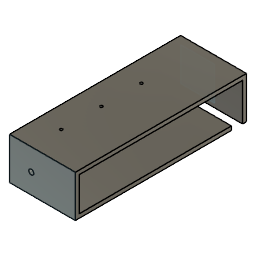
Final_3d_Model 1 (Autodesk Fusion 360 design; units mm, degrees)
part number: 2026-03-23-13-58-40-375
Autodesk Fusion 360 part; units mm, degrees
sketch "Sketch1" plane through (0, 0, 0) normal (0, 1, 0) x (1, 0, 0)
  line L0 (0, 0) -> (0, -42.3)
  line L1 (0, -42.3) -> (-42.3, -42.3)
  line L2 (-42.3, -42.3) -> (-42.3, 0)
  line L3 (-42.3, 0) -> (0, 0)
  line L4 (-42.3, -42.3) -> (-42.3, -52.3)
  line L5 (-42.3, -52.3) -> (-52.3, -52.3)
  line L6 (-52.3, -52.3) -> (10, -52.3)
  line L7 (10, -52.3) -> (10, 10)
  line L8 (10, 10) -> (-52.3, 10)
  line L9 (-52.3, 10) -> (-52.3, -52.3)
  dimension "d1" = 42.3
  dimension "d2" = 42.3
  dimension "d3" = 10
  dimension "d4" = 10
  constraint coincident L0.start L3.end
  constraint vertical L0
  constraint perpendicular L0 L1
  constraint perpendicular L1 L2
  constraint perpendicular L0 L3
  constraint perpendicular L1 L4
  constraint perpendicular L4 L5
  constraint horizontal L6
  constraint vertical L7
  constraint horizontal L8
  constraint vertical L9
  measures "d1" distance of L0.start L0.end
  measures "d2" distance of L0.end L1.end
  measures "d3" distance of L1.end L4.end
  measures "d4" distance of L4.end L5.end
extrude "Extrude1" add sketch "Sketch1" along normal blind 38.8 makes body 1
sketch "Sketch2" plane through (0, 0, 0) normal (0, 1, 0) x (1, 0, 0)
extrude "Extrude2" add 1 faces at (-28.2, 38.8, -6.6667) along direction (0, 1, 0) blind 10 on bodies 1 bodies 1
sketch "Sketch3" plane through (0, 0, 0) normal (0, 0, 1) x (-1, 0, 0)
  line L0 (42.3, 0) -> (0, 0)
  line L1 (0, 0) -> (0, -48.8)
  line L2 (0, -48.8) -> (42.3, -48.8)
  line L3 (42.3, -48.8) -> (42.3, 0)
  line L4 (42.3, -48.8) -> (0, -48.8)
  line L5 (0, -48.8) -> (0, -38.8)
  line L6 (0, -38.8) -> (42.3, -38.8)
  line L7 (42.3, -38.8) -> (42.3, -48.8)
  dimension "d9" = 10
  constraint horizontal L4
  constraint vertical L5
  constraint horizontal L6
  constraint vertical L7
  constraint coincident L2.end L3.start
  measures "d9" distance of L2.end L6.end
extrude "Extrude3" add sketch "Sketch3" along normal blind 52.3 contours L1 L2 L3 L4 L5 L6 L7 bodies 1
sketch "Sketch4" plane through (0, 38.8, 0) normal (0, -1, 0) x (1, 0, 0)
  line L0 (0, 42.3) -> (-42.3, 42.3)
  line L1 (-42.3, 42.3) -> (-42.3, 0)
  line L2 (-42.3, 0) -> (0, 0)
  line L3 (0, 0) -> (0, 42.3)
sketch "Sketch5" plane through (0, 0, 0) normal (0, 1, 0) x (1, 0, 0)
  circle A0 centre (-20, -20) radius 3
  dimension "d12" = 6
  measures "d12" diameter of A0
extrude "Extrude4" add sketch "Sketch5" against normal blind 250 separate body makes body 2
sketch "Sketch6" plane through (0, 0, 0) normal (0, 1, 0) x (1, 0, 0)
  line L0 (-28.6487, -14.9801) -> (-24.3014, -7.4901)
  line L1 (-11.3283, -15.0199) -> (-15.6412, -7.51)
  arc A0 (-15.6412, -7.51) -> (-24.3014, -7.4901) centre (-19.977, -10) ccw
  arc A1 (-28.6487, -14.9801) -> (-11.3283, -15.0199) centre (-20, -20) ccw
  constraint coincident A0.centre A1
  constraint tangent L0 A1
  constraint tangent L1 A0
  constraint tangent L1 A1
  constraint tangent L0 A0
extrude "Extrude5" add sketch "Sketch6" against normal blind 5 separate body makes body 3
sketch "Sketch7" plane through (0, -5, 0) normal (0, -1, 0) x (1, 0, 0)
  arc A0 (-11.3283, 15.0199) -> (-28.6487, 14.9801) centre (-20, 20) ccw
  line L0 (-28.6487, 14.9801) -> (-24.3014, 7.4901)
  arc A1 (-24.3014, 7.4901) -> (-15.6412, 7.51) centre (-19.977, 10) ccw
  line L1 (-15.6412, 7.51) -> (-11.3283, 15.0199)
  arc A2 (-9.5939, 14.0239) -> (-30.3785, 13.9761) centre (-20, 20) ccw
  line L2 (-30.3785, 13.9761) -> (-26.0312, 6.4861)
  arc A3 (-26.0312, 6.4861) -> (-13.9068, 6.514) centre (-19.977, 10) ccw
  line L3 (-13.9068, 6.514) -> (-9.5939, 14.0239)
  dimension "d17" = 2
extrude "Extrude6" add sketch "Sketch7" along normal blind 2 contours A0 L0 A1 L1 | A2 L2 A3 L3 bodies 3
sketch "Sketch8" plane through (0, 0, 0) normal (0, 1, 0) x (-1, 0, 0)
  arc A0 (28.6487, 14.9801) -> (11.3283, 15.0199) centre (20, 20) ccw
  line L0 (11.3283, 15.0199) -> (15.6412, 7.51)
  arc A1 (15.6412, 7.51) -> (24.3014, 7.4901) centre (19.977, 10) ccw
  line L1 (24.3014, 7.4901) -> (28.6487, 14.9801)
  arc A2 (30.3785, 13.9761) -> (9.5939, 14.0239) centre (20, 20) ccw
  line L2 (9.5939, 14.0239) -> (13.9068, 6.514)
  arc A3 (13.9068, 6.514) -> (26.0312, 6.4861) centre (19.977, 10) ccw
  line L3 (26.0312, 6.4861) -> (30.3785, 13.9761)
  dimension "d20" = 2
extrude "Extrude7" add sketch "Sketch8" along normal blind 2 contours A0 L0 A1 L1 | A2 L2 A3 L3 bodies 3
sketch "Sketch9" plane through (0, -7, 0) normal (0, -1, 0) x (1, 0, 0)
  line L0 (-13.9068, 6.514) -> (-9.5939, 14.0239)
  arc A0 (-9.5939, 14.0239) -> (-30.3785, 13.9761) centre (-20, 20) ccw
  line L1 (-30.3785, 13.9761) -> (-26.0312, 6.4861)
  arc A1 (-26.0312, 6.4861) -> (-13.9068, 6.514) centre (-19.977, 10) ccw
  circle A2 centre (-20, 20) radius 3
  constraint concentric A0 A2
extrude "Extrude8" cut sketch "Sketch9" against normal blind 19 contours A2 bodies 3
move_body "Move1" bodies 3 to x (1, 0, 0) y (0, 1, 0) z (0, 0, 1) at (0, -30, 0)
sketch "Sketch10" plane through (0, 0, 0) normal (0, 1, 0) x (1, 0, 0)
  circle A0 centre (-20, -35) radius 2.5
  dimension "d25" = 5
  measures "d25" diameter of A0
extrude "Extrude9" add sketch "Sketch10" along normal blind 5 separate body makes body 4
sketch "Sketch11" plane through (0, 0, 0) normal (0, 0, 1) x (1, 0, 0)
  circle A0 centre (-20, 2.5) radius 1.5
  dimension "d28" = 3
  measures "d28" diameter of A0
move_body "Move2" bodies 4 to x (1, 0, 0) y (0, 1, 0) z (0, 0, 1) at (0, 0, -50)
extrude "Extrude10" cut sketch "Sketch11" against normal blind 15 bodies 4
move_body "Move3" bodies 4 to x (1, 0, 0) y (0, 1, 0) z (0, 0, 1) at (0, 0, 50)
move_body "Move4" bodies 4 to x (1, 0, 0) y (0, 1, 0) z (0, 0, 1) at (0, -35, 0)
copy_body "CopyPasteBodies1" bodies 3 4 makes body 5 makes body 6
move_body "Move5" bodies 5 6 to x (1, 0, 0) y (0, 1, 0) z (0, 0, 1) at (0, -50, 0)
copy_body "CopyPasteBodies2" bodies 5 6 makes body 7 makes body 8
move_body "Move6" bodies 7 8 to x (1, 0, 0) y (0, 1, 0) z (0, 0, 1) at (0, -50, 0)
extrude "Extrude11" cut 1 faces at (-20.0747, -250, 19.1355) along direction (0, 1, 0) blind 100 on bodies 2 bodies 2
extrude "Extrude12" add 1 faces at (-20.0747, -150, 19.1355) along direction (0, -1, 0) blind 12 on bodies 2 bodies 2
sketch "Sketch12" plane through (0, 0, 0) normal (0, -1, 0) x (1, 0, 0)
  line L0 (-42.3, 0) -> (-42.3, 42.3)
  line L1 (-42.3, 42.3) -> (0, 42.3)
  line L2 (0, 42.3) -> (0, 0)
  line L3 (0, 0) -> (-42.3, 0)
  line L4 (-52.3, 52.3) -> (-52.3, -10)
  line L5 (-52.3, -10) -> (10, -10)
  line L6 (10, -10) -> (10, 52.3)
  line L7 (10, 52.3) -> (-52.3, 52.3)
  line L8 (0, 0) -> (10, 0)
  line L9 (0, 42.3) -> (10, 42.3)
  constraint coincident L2.end L3.start
  constraint coincident L6 L8.end
  constraint perpendicular L6 L8
  constraint coincident L1.end L2.start
  constraint coincident L6 L9.end
  constraint perpendicular L6 L9
extrude "Extrude13" add sketch "Sketch12" along normal blind 165 contours L0 L1 L3 L4 L5 L6 L7 L8 L9 bodies 1
sketch "Sketch13" plane through (0, 0, 52.3) normal (0, 0, 1) x (-1, 0, 0)
  line L0 (-10, -48.8) -> (52.3, -48.8)
  line L1 (52.3, -48.8) -> (52.3, 165)
  line L2 (52.3, 165) -> (-10, 165)
  line L3 (-10, 165) -> (-10, -48.8)
  line L4 (52.3, -48.8) -> (52.3, -38.8)
  line L5 (21.15, -38.8) -> (21.15, -33.8)
  line L6 (21.15, -33.8) -> (24.15, -33.8)
  line L7 (21.15, -33.8) -> (18.15, -33.8)
  line L8 (21.15, -38.8) -> (24.15, -38.8)
  line L9 (21.15, -38.8) -> (18.15, -38.8)
  line L10 (24.15, -38.8) -> (24.15, -33.8)
  line L11 (18.15, -38.8) -> (18.15, -33.8)
  dimension "d37" = 10
  dimension "d38" = 31.15
  dimension "d39" = 5
  dimension "d40" = 3
  dimension "d41" = 3
  dimension "d42" = 3
  dimension "d43" = 3
  constraint coincident L0.end L1.start
  constraint perpendicular L0 L4
  constraint perpendicular L5 L6
  constraint perpendicular L5 L7
  constraint perpendicular L5 L8
  constraint perpendicular L5 L9
  measures "d37" distance of L0.end L4.end
  measures "d38" distance of L4.end L5.start
  measures "d39" distance of L5.start L5.end
  measures "d40" distance of L5.end L6.end
  measures "d41" distance of L5.end L7.end
  measures "d42" distance of L5.start L8.end
  measures "d43" distance of L5.start L9.end
extrude "Extrude14" cut sketch "Sketch13" against normal blind 18 contours L5 L7 L9 L11 | L5 L6 L8 L10 bodies 1
extrude "Extrude15" cut 1 faces at (-20.15, 33.8, 48.9667) along direction (0, -1, 0) blind 2 on bodies 1 bodies 1
extrude "Extrude16" cut 1 faces at (-24.15, 36.4667, 48.9667) along direction (-1, 0, 0) blind 3 on bodies 1 bodies 1
extrude "Extrude17" cut 1 faces at (-18.15, 36.4667, 48.9667) along direction (1, 0, 0) blind 3 on bodies 1 bodies 1
extrude "Extrude18" cut 3 faces at (-20.3665, -132.9891, 35) (-20.3665, -82.9891, 35) (-20.334, -31.51, 35) along direction (0, 0, 1) blind 60 on bodies 4 6 8 bodies 1
sketch "Sketch14" plane through (0, -165, 0) normal (0, -1, 0) x (1, 0, 0)
  line L0 (10, 0) -> (-42.3, 0)
  line L1 (-42.3, 0) -> (-42.3, 42.3)
  line L2 (-42.3, 42.3) -> (10, 42.3)
  line L3 (10, 42.3) -> (10, 52.3)
  line L4 (10, 52.3) -> (-52.3, 52.3)
  line L5 (-52.3, 52.3) -> (-52.3, -10)
  line L6 (-52.3, -10) -> (10, -10)
  line L7 (10, -10) -> (10, 0)
  line L8 (-52.3, 52.3) -> (10, 52.3)
  line L9 (10, 52.3) -> (10, -10)
  line L10 (10, -10) -> (-52.3, -10)
  line L11 (-52.3, -10) -> (-52.3, 52.3)
  circle A0 centre (-20, 20) radius 3.125
  dimension "d54" = 6.25
  constraint horizontal L8
  constraint vertical L9
  constraint horizontal L10
  constraint vertical L11
  constraint coincident L6.end L7.start
  constraint coincident L4.end L5.start
  measures "d54" diameter of A0
extrude "Extrude19" add sketch "Sketch14" along normal blind 10 bodies 1
extrude "Extrude20" add 1 faces at (-23.15, 31.8, 45.6333) along direction (0, 1, 0) blind 7 on bodies 1 bodies 1
extrude "Extrude21" cut 1 faces at (-19.9046, -78, 10.0028) along direction (0, -1, 0) blind 2 on bodies 5 bodies 5
extrude "Extrude22" cut 1 faces at (-19.9046, -87, 10.0028) along direction (0, 1, 0) blind 2 on bodies 5 bodies 5
extrude "Extrude23" cut 1 faces at (-19.9046, -137, 10.0028) along direction (0, 1, 0) blind 2 on bodies 7 bodies 7
extrude "Extrude24" cut 1 faces at (-19.9046, -37, 10.0028) along direction (0, 1, 0) blind 2 on bodies 3 bodies 3
extrude "Extrude25" cut 1 faces at (-19.9046, -28, 10.0028) along direction (0, -1, 0) blind 2 on bodies 3 bodies 3
extrude "Extrude26" cut 1 faces at (-19.9046, -128, 10.0028) along direction (0, -1, 0) blind 2 on bodies 7 bodies 7
extrude "Extrude27" add 1 faces at (-19.9061, -130, 10.6695) along direction (0, 1, 0) blind 2.5 on bodies 7 bodies 7
extrude "Extrude28" add 1 faces at (-19.9061, -80, 10.6695) along direction (0, 1, 0) blind 2.5 on bodies 5 bodies 5
extrude "Extrude29" add 1 faces at (-19.9061, -30, 10.6695) along direction (0, 1, 0) blind 2.5 on bodies 3 bodies 3
extrude "Extrude30" add 1 faces at (-19.9061, -135, 10.6695) along direction (0, -1, 0) blind 2.5 on bodies 7 bodies 7
extrude "Extrude31" add 1 faces at (-19.9061, -85, 10.6695) along direction (0, -1, 0) blind 2.5 on bodies 5 bodies 5
extrude "Extrude32" add 1 faces at (-19.9061, -35, 10.6695) along direction (0, -1, 0) blind 2.5 on bodies 3 bodies 3
sketch "Sketch15" plane through (0, 0, -10) normal (0, 0, -1) x (1, 0, 0)
  line L0 (-52.3, 175) -> (-52.3, -48.8)
  line L1 (-52.3, -48.8) -> (10, -48.8)
  line L2 (10, -48.8) -> (10, 175)
  line L3 (10, 175) -> (-52.3, 175)
  line L4 (-50.3, -46.8) -> (8, -46.8)
  line L5 (8, -46.8) -> (8, 173)
  line L6 (8, 173) -> (-50.3, 173)
  line L7 (-50.3, 173) -> (-50.3, -46.8)
  line L8 (8, -46.8) -> (10, -46.8)
  line L9 (8, 173) -> (10, 173)
  dimension "d83" = -2
  constraint coincident L2 L8.end
  constraint perpendicular L2 L8
  constraint coincident L2 L9.end
  constraint perpendicular L2 L9
extrude "Extrude33" add sketch "Sketch15" along normal blind 50 contours L0 L1 L2 L3 L4 L6 L7 L8 L9 bodies 1
sketch "Sketch16" plane through (0, 0, -60) normal (0, 0, -1) x (1, 0, 0)
  line L0 (-50.3, 173) -> (10, 173)
  line L1 (10, 173) -> (10, 175)
  line L2 (10, 175) -> (-52.3, 175)
  line L3 (-52.3, 175) -> (-52.3, -48.8)
  line L4 (-52.3, -48.8) -> (10, -48.8)
  line L5 (10, -48.8) -> (10, -46.8)
  line L6 (10, -46.8) -> (-50.3, -46.8)
  line L7 (-50.3, -46.8) -> (-50.3, 173)
  line L8 (10, -48.8) -> (-52.3, -48.8)
  line L9 (-52.3, -48.8) -> (-52.3, 175)
  line L10 (-52.3, 175) -> (10, 175)
  line L11 (10, 175) -> (10, -48.8)
  constraint horizontal L8
  constraint vertical L9
  constraint horizontal L10
  constraint vertical L11
  constraint coincident L2.end L3.start
  constraint coincident L4.end L5.start
extrude "Extrude34" add sketch "Sketch16" along normal blind 5 separate body contours L0 L6 L7 L11 makes body 9
extrude "Extrude35" add 1 faces at (-10.1, 46.8, -61.6667) along direction (0, 1, 0) blind 2 on bodies 9 bodies 1 9
extrude "Extrude36" add 1 faces at (-30.2, -173, -63.3333) along direction (0, -1, 0) blind 2 on bodies 1 bodies 1
extrude "Extrude37" add 1 faces at (-50.3, -26.4667, -63.3333) along direction (-1, 0, 0) blind 2 on bodies 1 bodies 1
sketch "Sketch17" plane through (0, 0, -10) normal (0, 0, -1) x (1, 0, 0)
  line L0 (-50.3, -46.8) -> (10, -46.8)
  line L1 (10, -46.8) -> (10, 173)
  line L2 (10, 173) -> (-50.3, 173)
  line L3 (-50.3, 173) -> (-50.3, -46.8)
  line L4 (10, -46.8) -> (-20.15, -46.8)
  line L5 (-20.15, -46.8) -> (-20.15, -41.8)
  line L6 (-20.15, -41.8) -> (-15.15, -41.8)
  line L7 (-20.15, -41.8) -> (-25.15, -41.8)
  line L8 (-15.15, -41.8) -> (-15.15, 8.2)
  line L9 (-25.15, -41.8) -> (-25.15, 8.2)
  line L10 (-15.15, 8.2) -> (-25.15, 8.2)
  dimension "d94" = 30.15
  dimension "d95" = 5
  dimension "d96" = 5
  dimension "d97" = 5
  dimension "d98" = 50
  dimension "d99" = 50
  constraint coincident L0.end L1.start
  constraint perpendicular L1 L4
  constraint perpendicular L0 L5
  constraint perpendicular L5 L6
  constraint perpendicular L5 L7
  constraint perpendicular L6 L8
  constraint perpendicular L7 L9
  measures "d94" distance of L0.end L4.end
  measures "d95" distance of L4.end L5.end
  measures "d96" distance of L5.end L6.end
  measures "d97" distance of L5.end L7.end
  measures "d98" distance of L6.end L8.end
  measures "d99" distance of L7.end L9.end
extrude "Extrude38" cut sketch "Sketch17" against normal blind 5 contours L6 L7 L8 L9 L10 bodies 1
extrude "Extrude39" add 1 faces at (-18.4833, 41.8, -8.3333) along direction (0, -1, 0) blind 5 on bodies 1 bodies 1
extrude "Extrude40" cut 1 faces at (-21.8167, 6.8, -5) along direction (0, 0, 1) blind 15 on bodies 1 bodies 1
extrude "Extrude41" cut 1 faces at (-18.4833, 36.8, -6.6667) along direction (0, 1, 0) blind 2 on bodies 1 bodies 1
extrude "Extrude42" add 1 faces at (-50.3, -99.7333, -26.6667) along direction (1, 0, 0) blind 3 on bodies 1 bodies 1
extrude "Extrude43" add 1 faces at (-28.2, 46.8, -26.6667) along direction (0, -1, 0) blind 3 on bodies 1 bodies 1
extrude "Extrude44" add 1 faces at (-28.2, -173, -26.6667) along direction (0, 1, 0) blind 3 on bodies 1 bodies 1
extrude "Extrude45" cut 1 faces at (3.3333, 0, 14.1) along direction (0, 1, 0) blind 35 on bodies 1 bodies 1
extrude "Extrude46" add 1 faces at (-25.15, 23.1333, -6.6667) along direction (1, 0, 0) blind 10 on bodies 1 bodies 1
extrude "Extrude47" cut 1 faces at (3.3333, 35, 14.1) along direction (0, 1, 0) blind 10 on bodies 1 bodies 1
extrude "Extrude48" add 1 faces at (0, 42.9333, 28.2) along direction (1, 0, 0) blind 10 on bodies 1 bodies 1
sketch "Sketch18" plane through (10, 0, 0) normal (1, 0, 0) x (0, 1, 0)
  line L0 (38.8, 0) -> (-165, 0)
  line L1 (-165, 0) -> (-165, 42.3)
  line L2 (-165, 42.3) -> (38.8, 42.3)
  line L3 (38.8, 42.3) -> (38.8, 0)
  line L4 (-175, -65) -> (48.8, -65)
  line L5 (48.8, -65) -> (48.8, 52.3)
  line L6 (48.8, 52.3) -> (-175, 52.3)
  line L7 (-175, 52.3) -> (-175, -65)
  line L8 (-170, -60) -> (-170, -10)
  line L9 (-170, -10) -> (43.8, -10)
  line L10 (43.8, -10) -> (43.8, -60)
  line L11 (43.8, -60) -> (-170, -60)
  line L12 (38.8, 0) -> (38.8, -10)
  line L13 (0, 0) -> (0, -10)
  constraint coincident L0.start L3.end
  constraint coincident L9 L12.end
  constraint perpendicular L9 L12
  constraint coincident L13.start origin
  constraint coincident L9 L13.end
  constraint perpendicular L9 L13
extrude "Extrude49" cut sketch "Sketch18" against normal blind 20 contours L0 L9 L12 L13 | L0 L1 L2 L3 bodies 1
extrude "Extrude50" cut 1 faces at (-10, 25.8667, -6.6667) along direction (-1, 0, 0) blind 2 on bodies 1 bodies 1
extrude "Extrude51" cut 1 faces at (-12, 25.8667, -6.6667) along direction (-1, 0, 0) blind 15 on bodies 1 bodies 1
extrude "Extrude52" add 1 faces at (-2.3333, 0, -3.3333) along direction (0, 1, 0) blind 25 on bodies 1 bodies 1
extrude "Extrude53" add 1 faces at (-31.5333, -99.7333, -65) along direction (0, 0, -1) blind 100 on bodies 1 bodies 1
extrude "Extrude54" cut 1 faces at (-28.2, -98.7333, -60) along direction (0, 0, -1) blind 100 on bodies 1 bodies 1
extrude "Extrude55" add 11 faces at (10, 47.4667, -95) (10, -25.8, 48.9667) (10, -173.6667, -95) (10, -27.4667, -163.3333) (10, 45.8, -26.6667) (10, -171.6667, 45.6333) (10, -173.6667, -26.6667) (10, -170, -3.3333) (10, -168.3333, 28.2) (10, -172, -26.6667) (10, -46.6667, -6.6667) along direction (1, 0, 0) blind 25 on bodies 1 bodies 1
sketch "Sketch19" plane through (35, 0, 0) normal (1, 0, 0) x (0, 1, 0)
  line L0 (48.8, -165) -> (48.8, 52.3)
  line L1 (48.8, 52.3) -> (-175, 52.3)
  line L2 (-175, 52.3) -> (-175, -165)
  line L3 (-175, -165) -> (48.8, -165)
  line L4 (43.8, -10) -> (43.8, -160)
  line L5 (43.8, -160) -> (-170, -160)
  line L6 (-170, -160) -> (-170, -10)
  line L7 (-170, -10) -> (25, -10)
  line L8 (25, -10) -> (25, 0)
  line L9 (25, 0) -> (-165, 0)
  line L10 (-165, 0) -> (-165, 42.3)
  line L11 (-165, 42.3) -> (38.8, 42.3)
  line L12 (38.8, 42.3) -> (38.8, -10)
  line L13 (38.8, -10) -> (43.8, -10)
  line L14 (-165, 0) -> (-165, -10)
  constraint coincident L9.end L10.start
  constraint coincident L7 L14.end
  constraint perpendicular L7 L14
extrude "Extrude56" cut sketch "Sketch19" against normal blind 25 contours L7 L8 L9 L14 bodies 1
extrude "Extrude57" cut 1 faces at (-23.2, -99.7333, -165) along direction (0, 0, 1) blind 160 on bodies 1 bodies 1
extrude "Extrude58" add 1 faces at (10, -101.6667, -1.6667) along direction (1, 0, 0) blind 25 on bodies 1 bodies 1
extrude "Extrude59" cut 1 faces at (-12.2788, 22.1755, 52.3) along direction (0, 0, -1) blind 5 on bodies 1 bodies 1
extrude "Extrude60" cut 1 faces at (17.7083, -175, 20.7667) along direction (0, 1, 0) blind 5 on bodies 1 bodies 1
extrude "Extrude61" cut 1 faces at (5.9, 48.8, 12.4333) along direction (0, -1, 0) blind 5 on bodies 1 bodies 1
extrude "Extrude62" cut 1 faces at (-52.3, -98.7333, 29.8667) along direction (1, 0, 0) blind 5 on bodies 1 bodies 1
sketch "Sketch20" plane through (0, 38.8, 0) normal (0, -1, 0) x (1, 0, 0)
  circle A0 centre (-20, 20) radius 12.5
  dimension "d150" = 25
  measures "d150" diameter of A0
extrude "Extrude63" cut sketch "Sketch20" against normal blind 20 bodies 1
sketch "Sketch21" plane through (0, 0, 47.3) normal (0, 0, 1) x (-1, 0, 0)
  line L0 (47.3, -43.8) -> (47.3, 170)
  line L1 (47.3, 170) -> (-35, 170)
  line L2 (-35, 170) -> (-35, -43.8)
  line L3 (-35, -43.8) -> (47.3, -43.8)
  circle A0 centre (20, 82.5) radius 1.5
  circle A1 centre (20, 132.5) radius 1.5
  circle A2 centre (20, 32.5) radius 1.5
  circle A3 centre (20, 32.5) radius 1.625
  circle A4 centre (20, 82.5) radius 1.625
  circle A5 centre (20, 132.5) radius 1.625
  dimension "d153" = 3.25
  dimension "d154" = 3.25
  dimension "d155" = 3.25
  constraint concentric A2 A3
  constraint concentric A0 A4
  constraint concentric A1 A5
  measures "d153" diameter of A3
  measures "d154" diameter of A4
  measures "d155" diameter of A5
extrude "Extrude64" cut sketch "Sketch21" against normal blind 5 contours A3 | A4 | A5 bodies 1
sketch "Sketch22" plane through (0, -170, 0) normal (0, -1, 0) x (1, 0, 0)
  line L0 (-47.3, 47.3) -> (-47.3, -5)
  line L1 (-47.3, -5) -> (35, -5)
  line L2 (35, -5) -> (35, 47.3)
  line L3 (35, 47.3) -> (-47.3, 47.3)
  circle A0 centre (-20, 20) radius 3.125
hidden bodies 2
